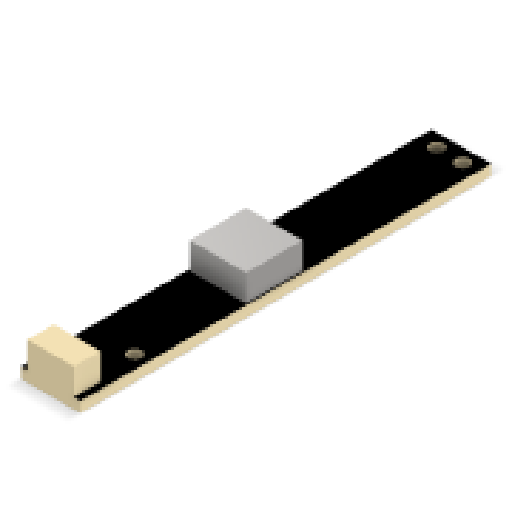
# Autodesk Inventor part: Waveshare OV5640
Saved by Autodesk Inventor 2023.2 (Build 272271000, 271)
## iProperties
Created: 2023-02-26
Part Number: Waveshare OV5640
Material: Aluminum 6061
Document SubType Name: Modeling
Designer: remop
Density: 2.7 g/cm^3
Appearance: Anodized - Black
Author: remop
Autodesk Inventor part; units mm, degrees
ref_plane "YZ Plane" through (0, 0, 0) normal (1, 0, 0) x (0, 1, 0)
ref_plane "XZ Plane" through (0, 0, 0) normal (0, 1, 0) x (-1, 0, 0)
ref_plane "XY Plane" through (0, 0, 0) normal (0, 0, 1) x (1, 0, 0)
sketch "Sketch1" plane through (0, 0, 0) normal (0, 1, 0) x (-1, 0, 0)
  line L0 (-4.5, -31) -> (4.5, -31)
  line L1 (4.5, -31) -> (4.5, 31)
  line L2 (4.5, 31) -> (-4.5, 31)
  line L3 (-4.5, 31) -> (-4.5, -31)
  line L4 (-4.5, -31) -> (4.5, 31) construction
  line L5 (4.5, -31) -> (-4.5, 31) construction
  circle A0 centre (-2.5, 20.8) radius 1.05
  circle A1 centre (-2.25, -29) radius 1.05
  circle A2 centre (1.75, -29) radius 1.05
  point P0 (0, 0)
  dimension "d0" = 62
  dimension "d1" = 9
  dimension "d2" = 2.1
  dimension "d3" = 2.75
  dimension "d4" = 4
  dimension "d5" = 2
  dimension "d6" = 49.8
  dimension "d7" = 2
  constraints: 12 end point, 3 centre point, 2 equal radius, 2 midpoint, 2 parallel, 1 horizontal, 1 horizontal alignment, 1 perpendicular
  measures "d0" distance of L0.end L1.end
  measures "d1" distance of L1.end L2.end
  measures "d2" diameter of A0
  measures "d3" distance from line of L1 A2.centre
  measures "d4" distance of A2.centre A1.centre
  measures "d5" distance from line of L3 A0.centre
  measures "d6" vertical distance of A1.centre A0.centre
  measures "d7" distance from line of L0 A1.centre
extrude "Extrusion1" add sketch "Sketch1" along normal blind 1.6
sketch "Sketch2" plane through (0, 1.6, 0) normal (0, 1, 0) x (1, 0, 0)
  line L0 (-4.5, 31) -> (-4.5, -31) projected
  line L1 (-4.5, -31) -> (4.5, -31) projected
  line L2 (4.5, -31) -> (4.5, 31) projected
  line L3 (4.5, 31) -> (-4.5, 31) projected
  circle A0 centre (2.5, -20.8) radius 1.05 projected
  circle A1 centre (2.25, 29) radius 1.05 projected
  circle A2 centre (-1.75, 29) radius 1.05 projected
  line L4 (4.25, -5.75) -> (-4.25, -5.75)
  line L5 (-4.25, -5.75) -> (-4.25, 2.75)
  line L6 (-4.25, 2.75) -> (4.25, 2.75)
  line L7 (4.25, 2.75) -> (4.25, -5.75)
  line L8 (4.25, -5.75) -> (-4.25, 2.75) construction
  line L9 (-4.25, -5.75) -> (4.25, 2.75) construction
  line L10 (-4.5, -31) -> (4.5, -31) projected
  line L11 (-3.5, -31) -> (3.5, -31)
  line L12 (3.5, -31) -> (3.5, -27)
  line L13 (3.5, -27) -> (-3.5, -27)
  line L14 (-3.5, -27) -> (-3.5, -31)
  point P0 (0, 0)
  point P1 (0, -1.5)
  point P2 (-3.5, -29)
  dimension "d10" = 8.5
  dimension "d11" = 29.5
  dimension "d12" = 1
  dimension "d13" = 1
  dimension "d14" = 4
  constraints: 20 end point, 4 parallel, 3 midpoint, 3 perpendicular, 2 horizontal, 1 point on line, 1 vertical alignment
  measures "d10" distance of L5.end L6.end
  measures "d11" distance from line of L1 point (0, -1.5)
  measures "d12" distance from line of L0 point (-3.5, -29)
  measures "d13" distance between parallel lines of L2 L12
  measures "d14" distance of L11.end L12.end
extrude "Extrusion2" add sketch "Sketch2" along normal blind 4 contours L14 L13 L12 L1 | L4 L5 L6 L7
equation "\"d13\" = d12"
body "Solid1"
